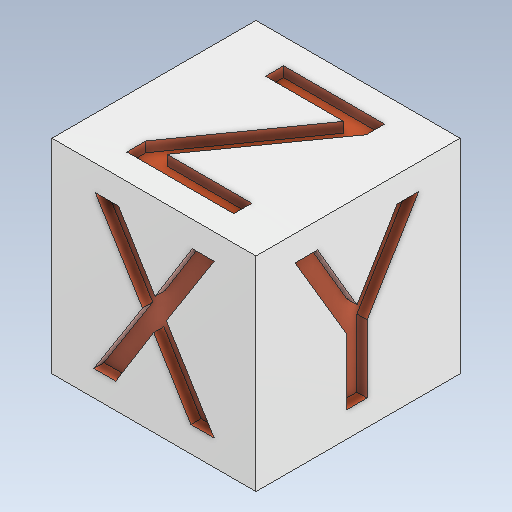
# Autodesk Inventor part: Cubo-0001-002
Saved by Autodesk Inventor 2025.2 (Build 292293000, 293)
## iProperties
Created: 2025-01-18
Part Number: Cubo-0001-002
Material: ABS plástico
Document SubType Name: Modeling
Designer: Gustavo Sousa
Density: 1.06 g/cm^3
Appearance: Suave - Branco
Author: Gustavo Sousa
Autodesk Inventor part; units mm, degrees
ref_plane "YZ Plane" through (0, 0, 0) normal (1, 0, 0) x (0, 1, 0)
ref_plane "XZ Plane" through (0, 0, 0) normal (0, 1, 0) x (-1, 0, 0)
ref_plane "XY Plane" through (0, 0, 0) normal (0, 0, 1) x (1, 0, 0)
sketch "Esboço1" plane through (0, 0, 0) normal (0, 0, 1) x (1, 0, 0)
  line L0 (-10, -10) -> (10, -10)
  line L1 (10, -10) -> (10, 10)
  line L2 (10, 10) -> (-10, 10)
  line L3 (-10, 10) -> (-10, -10)
  line L4 (-10, -10) -> (10, 10) construction
  line L5 (10, -10) -> (-10, 10) construction
  point P0 (0, 0)
  dimension "d0" = 20
  dimension "d1" = 20
  constraints: 12 end point, 2 midpoint, 2 parallel, 1 horizontal, 1 perpendicular
  measures "d0" distance of L2.end L1.end
  measures "d1" distance of L1.end L0.end
extrude "Extrusão1" add sketch "Esboço1" along normal mid plane 20
sketch "Esboço2" plane through (0, 0, 10) normal (0, 0, 1) x (1, 0, 0)
  line L0 (-10, 10) -> (10, 10) construction
  line L1 (10, 10) -> (10, -10) construction
  line L2 (10, -10) -> (-10, -10) construction
  line L3 (-10, -10) -> (-10, 10) construction
  line L4 (5.9015, -7.5) -> (3.6163, -7.5)
  line L5 (3.6163, -7.5) -> (-0.0304, -1.5194)
  line L6 (-0.0304, -1.5194) -> (-3.75, -7.5)
  line L7 (-3.75, -7.5) -> (-5.9015, -7.5)
  line L8 (-5.9015, -7.5) -> (-1.1244, 0.0122)
  line L9 (-1.1244, 0.0122) -> (-5.7557, 7.5)
  line L10 (-5.7557, 7.5) -> (-3.4704, 7.5)
  line L11 (-3.4704, 7.5) -> (0.1033, 1.6288)
  line L12 (0.1033, 1.6288) -> (3.75, 7.5)
  line L13 (3.75, 7.5) -> (5.9015, 7.5)
  line L14 (5.9015, 7.5) -> (1.2095, 0.1094)
  line L15 (1.2095, 0.1094) -> (5.9015, -7.5)
  point P0 (0, 0)
  constraints: 2 horizontal, 2 vertical, 2 other
extrude "Extrusão2" cut sketch "Esboço2" against normal blind 1
sketch "Esboço3" plane through (10, -10, 10) normal (1, 0, 0) x (0, 0, -1)
  line L0 (0, 20) -> (20, 20) construction
  line L1 (20, 20) -> (20, 0) construction
  line L2 (20, 0) -> (0, 0) construction
  line L3 (0, 0) -> (0, 20) construction
  line L4 (15.9562, 17.5) -> (10.8874, 9.137)
  line L5 (10.8874, 9.137) -> (10.8874, 2.5)
  line L6 (10.8874, 2.5) -> (8.8938, 2.5)
  line L7 (8.8938, 2.5) -> (8.8938, 8.9303)
  line L8 (8.8938, 8.9303) -> (3.825, 17.5)
  line L9 (3.825, 17.5) -> (6.0373, 17.5)
  line L10 (6.0373, 17.5) -> (9.9028, 10.8995)
  line L11 (9.9028, 10.8995) -> (13.8412, 17.5)
  line L12 (13.8412, 17.5) -> (15.9562, 17.5)
  point P0 (10, 10)
  constraints: 2 horizontal, 2 vertical, 2 other
extrude "Extrusão3" cut sketch "Esboço3" against normal blind 1
sketch "Esboço4" plane through (-10, 10, 10) normal (0, 1, 0) x (1, 0, 0)
  line L0 (0, 20) -> (20, 20) construction
  line L1 (20, 20) -> (20, 0) construction
  line L2 (20, 0) -> (0, 0) construction
  line L3 (0, 0) -> (0, 20) construction
  line L4 (15.3181, 2.5) -> (4.84, 2.5)
  line L5 (4.84, 2.5) -> (4.84, 4.3598)
  line L6 (4.84, 4.3598) -> (12.8626, 15.7253)
  line L7 (12.8626, 15.7253) -> (5.2046, 15.7253)
  line L8 (5.2046, 15.7253) -> (5.2046, 17.5)
  line L9 (5.2046, 17.5) -> (15.1114, 17.5)
  line L10 (15.1114, 17.5) -> (15.1114, 15.701)
  line L11 (15.1114, 15.701) -> (7.0036, 4.2747)
  line L12 (7.0036, 4.2747) -> (15.3181, 4.2747)
  line L13 (15.3181, 4.2747) -> (15.3181, 2.5)
  point P0 (10, 10)
  constraints: 2 horizontal, 2 vertical, 2 other
extrude "Extrusão4" cut sketch "Esboço4" against normal blind 1
